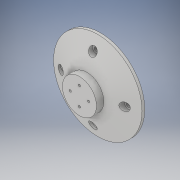
# Autodesk Inventor part: foot
Saved by Autodesk Inventor 2019 (Build 230136000, 136)
## iProperties
Created: 2024-08-06
Part Number: foot
Material: Generisch
Document SubType Name: Modeling
Designer: nic
Density: 1 g/cm^3
Appearance: Vorgabe
Author: nic
Autodesk Inventor part; units mm, degrees
ref_plane "YZ Plane" through (0, 0, 0) normal (1, 0, 0) x (0, 1, 0)
ref_plane "XZ Plane" through (0, 0, 0) normal (0, 1, 0) x (-1, 0, 0)
ref_plane "XY Plane" through (0, 0, 0) normal (0, 0, 1) x (1, 0, 0)
sketch "Skizze1" plane through (0, 0, 0) normal (0, 0, 1) x (1, 0, 0)
  circle A0 centre (0, 0) radius 75
  line L0 (0, 0) -> (13.5, 0) construction
  line L1 (13.5, 0) -> (-13.5, 0) construction
  line L2 (0, 0) -> (0, -13.5) construction
  line L3 (0, -13.5) -> (0, 13.5) construction
  circle A1 centre (0, 13.5) radius 1.6
  circle A2 centre (13.5, 0) radius 1.6
  circle A3 centre (0, -13.5) radius 1.6
  circle A4 centre (-13.5, 0) radius 1.6
  dimension "d0" = 150
  dimension "d1" = 13.5
  dimension "d2" = 27
  dimension "d3" = 13.5
  dimension "d4" = 27
  dimension "d5" = 3.2
  dimension "d6" = 3.2
  dimension "d7" = 3.2
  dimension "d8" = 3.2
  constraints: 8 end point, 5 centre point, 5 coincident, 2 point on line, 1 horizontal, 1 vertical
  measures "d0" diameter of A0
  measures "d1" distance of L0.start L0.end
  measures "d2" distance of L0.end L1.end
  measures "d3" distance of L0.start L2.end
  measures "d4" distance of L2.end L3.end
  measures "d5" diameter of A1
  measures "d6" diameter of A2
  measures "d7" diameter of A3
  measures "d8" diameter of A4
extrude "Extrusion1" add sketch "Skizze1" along normal blind 21
sketch "Skizze2" plane through (0, 0, 0) normal (0, 0, -1) x (-1, 0, 0)
  circle A0 centre (13.5, 0) radius 1.6 projected
  circle A1 centre (0, -13.5) radius 1.6 projected
  circle A2 centre (-13.5, 0) radius 1.6 projected
  circle A3 centre (0, 13.5) radius 1.6 projected
  circle A4 centre (0, 0) radius 75 projected
  circle A5 centre (13.5, 0) radius 1.6 projected
  line L0 (16, 2.5) -> (11, 2.5)
  line L1 (11, 2.5) -> (11, -2.5)
  line L2 (11, -2.5) -> (16, -2.5)
  line L3 (16, -2.5) -> (16, 2.5)
  line L4 (16, 2.5) -> (11, -2.5) construction
  line L5 (11, 2.5) -> (16, -2.5) construction
  line L6 (2.5, 16) -> (-2.5, 16)
  line L7 (-2.5, 16) -> (-2.5, 11)
  line L8 (-2.5, 11) -> (2.5, 11)
  line L9 (2.5, 11) -> (2.5, 16)
  line L10 (2.5, 16) -> (-2.5, 11) construction
  line L11 (-2.5, 16) -> (2.5, 11) construction
  line L12 (-11, 2.5) -> (-16, 2.5)
  line L13 (-16, 2.5) -> (-16, -2.5)
  line L14 (-16, -2.5) -> (-11, -2.5)
  line L15 (-11, -2.5) -> (-11, 2.5)
  line L16 (-11, 2.5) -> (-16, -2.5) construction
  line L17 (-16, 2.5) -> (-11, -2.5) construction
  line L18 (2.5, -11) -> (-2.5, -11)
  line L19 (-2.5, -11) -> (-2.5, -16)
  line L20 (-2.5, -16) -> (2.5, -16)
  line L21 (2.5, -16) -> (2.5, -11)
  line L22 (2.5, -11) -> (-2.5, -16) construction
  line L23 (-2.5, -11) -> (2.5, -16) construction
  dimension "d11" = 5
  dimension "d12" = 5
  dimension "d13" = 5
  dimension "d14" = 5
  dimension "d15" = 5
  dimension "d16" = 5
  dimension "d17" = 5
  dimension "d18" = 5
  constraints: 48 end point, 8 midpoint, 8 parallel, 4 horizontal, 4 perpendicular
  measures "d11" distance of L2.end L1.end
  measures "d12" distance of L1.end L0.end
  measures "d13" distance of L8.end L7.end
  measures "d14" distance of L7.end L6.end
  measures "d15" distance of L14.end L13.end
  measures "d16" distance of L13.end L12.end
  measures "d17" distance of L20.end L19.end
  measures "d18" distance of L19.end L18.end
extrude "Extrusion2" cut sketch "Skizze2" against normal blind 4 contours L3 L2 L1 L0 | L9 L8 L7 L6 | L15 L14 L13 L12 | L21 L20 L19 L18
draft "Flächenverjüngung1" angle -68 pull direction (0, 0, -1) faces at (-33.9595, -66.8711, 14) fixed edges at (-75, 0, 0)
sketch "Skizze3" plane through (0, 0, 21) normal (0, 0, 1) x (1, 0, 0)
  circle A0 centre (0, 0) radius 75 projected
  circle A1 centre (0, 0) radius 65
  dimension "d22" = 10
  constraints: 1 centre point
  measures "d22" radial gap between concentric circles of A0 A1
extrude "Extrusion3" cut sketch "Skizze3" against normal through all
sketch "Skizze4" plane through (0, 0, 21) normal (0, 0, 1) x (1, 0, 0)
  circle A0 centre (0, 0) radius 25
  circle A1 centre (-13.5, 0) radius 1.6 projected
  circle A2 centre (0, -13.5) radius 1.6 projected
  circle A3 centre (13.5, 0) radius 1.6 projected
  circle A4 centre (0, 13.5) radius 1.6 projected
  dimension "d25" = 50
  constraints: 1 centre point, 1 coincident
  measures "d25" diameter of A0
extrude "Extrusion4" add sketch "Skizze4" against normal blind 5
sketch "Skizze5" plane through (0, 0, 21) normal (0, 0, 1) x (1, 0, 0)
  circle A0 centre (0, 0) radius 25 projected
  circle A1 centre (-13.5, 0) radius 1.6 projected
  circle A2 centre (0, -13.5) radius 1.6 projected
  circle A3 centre (13.5, 0) radius 1.6 projected
  circle A4 centre (0, 13.5) radius 1.6 projected
extrude "Extrusion5" add sketch "Skizze5" along normal blind 10
sketch "Skizze6" plane through (0, 0, 0) normal (0, 0, -1) x (-1, 0, 0)
  line L0 (16.5, -16.5) -> (-16.5, -16.5)
  line L1 (-16.5, -16.5) -> (-16.5, 16.5)
  line L2 (-16.5, 16.5) -> (16.5, 16.5)
  line L3 (16.5, 16.5) -> (16.5, -16.5)
  line L4 (16.5, -16.5) -> (-16.5, 16.5) construction
  line L5 (-16.5, -16.5) -> (16.5, 16.5) construction
  point P0 (0, 0)
  dimension "d30" = 33
  dimension "d31" = 33
  constraints: 12 end point, 2 midpoint, 2 parallel, 1 horizontal, 1 perpendicular
  measures "d30" distance of L1.end L2.end
  measures "d31" distance of L0.end L1.end
extrude "Extrusion6" cut sketch "Skizze6" against normal blind 12
sketch "Skizze7" plane through (0, 0, 31) normal (0, 0, 1) x (1, 0, 0)
  circle A0 centre (0, 0) radius 47.044
  circle A1 centre (0, -47.044) radius 3.15
  circle A2 centre (47.044, 0) radius 3.15
  circle A3 centre (0, 47.044) radius 3.15
  circle A4 centre (-47.044, 0) radius 3.15
  dimension "d34" = 6.3
  dimension "d37" = 360
  constraints: 4 centre point, 1 coincident, 1 vertical alignment, 11 other
  measures "d34" diameter of A1
extrude "Extrusion7" cut sketch "Skizze7" against normal through all contours A0 A2 | A0 A2 | A3 A0 | A0 A3 | A1 A0 | A0 A1 | A4 A0 | A0 A4
sketch "Skizze8" plane through (0, 0, 31) normal (0, 0, 1) x (1, 0, 0)
  spline S0 degree 5 poles (-43.894, 0) (-43.894, 0.3302) (-43.9373, 0.6608) (-44.0238, 0.9696) (-44.1378, 1.248) (-44.4172, 1.7647) (-44.585, 1.9986) (-44.7684, 2.2019) (-44.9622, 2.3774) (-45.4726, 2.7569) (-45.7996, 2.9275) (-46.1378, 3.0471) (-46.4823, 3.1191) (-47.3034, 3.1749) (-47.7826, 3.118) (-48.2572, 2.9717) (-48.7217, 2.7241) (-49.3483, 2.1659) (-49.5453, 1.9493) (-49.7259, 1.6974) (-49.8813, 1.4099) (-50.073, 0.8908) (-50.1322, 0.6786) (-50.1732, 0.4563) (-50.194, 0.2281) (-50.194, -0.2281) (-50.1732, -0.4563) (-50.1322, -0.6786) (-50.073, -0.8908) (-49.8813, -1.4099) (-49.7259, -1.6974) (-49.5453, -1.9493) (-49.3483, -2.1659) (-48.7217, -2.7241) (-48.2572, -2.9717) (-47.7826, -3.118) (-47.3034, -3.1749) (-46.4805, -3.119) (-46.1343, -3.0464) (-45.7943, -2.9257) (-45.4658, -2.7534) (-44.9547, -2.3708) (-44.7615, -2.1948) (-44.5788, -1.9909) (-44.4117, -1.7565) (-44.1346, -1.2402) (-44.022, -0.9631) (-43.9367, -0.6562) (-43.894, -0.3278) (-43.894, 0) knots 0 0 0 0 0 0 0.065094 0.065094 0.065094 0.065094 0.134372 0.134372 0.134372 0.134372 0.239898 0.239898 0.239898 0.239898 0.383319 0.383319 0.383319 0.383319 0.45503 0.45503 0.45503 0.45503 0.500006 0.500006 0.500006 0.500006 0.544983 0.544983 0.544983 0.544983 0.616692 0.616692 0.616692 0.616692 0.760109 0.760109 0.760109 0.760109 0.866177 0.866177 0.866177 0.866177 0.935362 0.935362 0.935362 0.935362 1 1 1 1 1 1 projected
  spline S1 degree 5 poles (3.15, -47.044) (3.15, -46.5444) (3.051, -46.0483) (2.8557, -45.5691) (2.5553, -45.1095) (1.9343, -44.5455) (1.7275, -44.3902) (1.4934, -44.2493) (1.2314, -44.1292) (0.7704, -43.9842) (0.5868, -43.9403) (0.3957, -43.9099) (0.2003, -43.8943) (-0.325, -43.8935) (-0.6557, -43.9362) (-0.9647, -44.0222) (-1.2433, -44.1358) (-1.7606, -44.4145) (-1.9947, -44.5819) (-2.1984, -44.7649) (-2.3741, -44.9584) (-2.7558, -45.47) (-2.9276, -45.7988) (-3.0478, -46.139) (-3.1198, -46.4853) (-3.1744, -47.3066) (-3.1173, -47.7839) (-2.9715, -48.2566) (-2.7251, -48.7192) (-2.1695, -49.3449) (-1.9533, -49.5422) (-1.7017, -49.7232) (-1.4144, -49.8791) (-0.8957, -50.0715) (-0.6835, -50.1311) (-0.4613, -50.1725) (-0.2331, -50.1936) (0.2251, -50.1944) (0.4555, -50.1736) (0.6798, -50.1321) (0.8939, -50.0721) (1.4121, -49.8799) (1.6976, -49.7254) (1.9479, -49.5461) (2.1633, -49.3505) (2.6888, -48.7626) (2.9252, -48.3431) (3.0756, -47.9126) (3.15, -47.4768) (3.15, -47.044) knots 0 0 0 0 0 0 0.15092 0.15092 0.15092 0.15092 0.21412 0.21412 0.21412 0.21412 0.25264 0.25264 0.25264 0.25264 0.317704 0.317704 0.317704 0.317704 0.386937 0.386937 0.386937 0.386937 0.493038 0.493038 0.493038 0.493038 0.635903 0.635903 0.635903 0.635903 0.707661 0.707661 0.707661 0.707661 0.752636 0.752636 0.752636 0.752636 0.798003 0.798003 0.798003 0.798003 0.869251 0.869251 0.869251 0.869251 1 1 1 1 1 1 projected
  spline S2 degree 5 poles (3.15, 47.044) (3.15, 47.4768) (3.0756, 47.9125) (2.9252, 48.3431) (2.6888, 48.7626) (2.1633, 49.3505) (1.9479, 49.5461) (1.6976, 49.7254) (1.4121, 49.8799) (0.8957, 50.0715) (0.6835, 50.1311) (0.4613, 50.1725) (0.2331, 50.1936) (-0.2251, 50.1944) (-0.4555, 50.1736) (-0.6798, 50.1321) (-0.8939, 50.0721) (-1.4144, 49.8791) (-1.7017, 49.7232) (-1.9533, 49.5422) (-2.1695, 49.3449) (-2.7251, 48.7192) (-2.9715, 48.2566) (-3.1173, 47.7839) (-3.1744, 47.3066) (-3.1198, 46.4853) (-3.0478, 46.139) (-2.9276, 45.7988) (-2.7558, 45.47) (-2.3741, 44.9584) (-2.1984, 44.7649) (-1.9947, 44.5819) (-1.7606, 44.4145) (-1.2448, 44.1366) (-0.968, 44.0236) (-0.6613, 43.9378) (-0.333, 43.8945) (0.1924, 43.8937) (0.3899, 43.9089) (0.583, 43.9394) (0.7686, 43.9836) (1.2314, 44.1292) (1.4934, 44.2493) (1.7275, 44.3902) (1.9343, 44.5455) (2.5553, 45.1095) (2.8558, 45.5692) (3.051, 46.0483) (3.15, 46.5444) (3.15, 47.044) knots 0 0 0 0 0 0 0.130746 0.130746 0.130746 0.130746 0.201993 0.201993 0.201993 0.201993 0.246967 0.246967 0.246967 0.246967 0.292334 0.292334 0.292334 0.292334 0.364091 0.364091 0.364091 0.364091 0.506958 0.506958 0.506958 0.506958 0.613059 0.613059 0.613059 0.613059 0.682292 0.682292 0.682292 0.682292 0.746965 0.746965 0.746965 0.746965 0.785877 0.785877 0.785877 0.785877 0.849079 0.849079 0.849079 0.849079 1 1 1 1 1 1 projected
  spline S3 degree 2 poles (50.194, 0) (50.194, 5.456) (45.469, 2.728) (40.744, 0) (45.469, -2.728) (50.194, -5.456) (50.194, 0) knots 0 0 0 0.333333 0.333333 0.666667 0.666667 1 1 1 weights 1 0.5 1 0.5 1 0.5 1 projected
  circle A0 centre (0, -47.044) radius 3.15 projected
  circle A1 centre (0, -47.044) radius 6
  circle A2 centre (-47.044, 0) radius 3.15 projected
  circle A3 centre (-47.044, 0) radius 6
  circle A4 centre (0, 47.044) radius 3.15 projected
  circle A5 centre (0, 47.044) radius 6
  circle A6 centre (46.8331, 0) radius 6
  point P0 (0, 0)
  dimension "d41" = 12
  dimension "d42" = 12
  dimension "d43" = 12
  dimension "d44" = 12
  constraints: 4 centre point, 3 coincident, 7 other
  measures "d41" diameter of A1
  measures "d42" diameter of A3
  measures "d43" diameter of A5
  measures "d44" diameter of A6
extrude "Extrusion8" cut sketch "Skizze8" against normal blind 25 contours S1 | A1 | A3 | A5 | A6
